Autodesk Fusion 360 part; units mm, degrees
(part 10 of 11)
  spline S69 degree 5 poles (7.9623, -22.9033) (7.9606, -22.9006) (7.9574, -22.8954) (7.9525, -22.8875) (7.9459, -22.8771) (7.9377, -22.8641) (7.9294, -22.8512) (7.9211, -22.8383) (7.9127, -22.8255) (7.9043, -22.8127) (7.8959, -22.8) (7.8874, -22.7874) (7.8788, -22.7748) (7.8702, -22.7623) (7.8616, -22.7498) (7.8529, -22.7374) (7.8442, -22.725) (7.8354, -22.7128) (7.8266, -22.7005) (7.8178, -22.6884) (7.8089, -22.6763) (7.7999, -22.6643) (7.7909, -22.6523) (7.7819, -22.6404) (7.7728, -22.6286) (7.7637, -22.6168) (7.7545, -22.6051) (7.7453, -22.5935) (7.7361, -22.5819) (7.7268, -22.5704) (7.7174, -22.559) (7.708, -22.5476) (7.6986, -22.5363) (7.6891, -22.5251) (7.6795, -22.5139) (7.6699, -22.5029) (7.6603, -22.4919) (7.6506, -22.481) (7.6409, -22.4701) (7.6311, -22.4593) (7.6213, -22.4486) (7.6114, -22.438) (7.6015, -22.4275) (7.5915, -22.417) (7.5815, -22.4067) (7.5715, -22.3964) (7.5613, -22.3862) (7.5512, -22.376) (7.5409, -22.366) (7.5307, -22.3561) (7.5204, -22.3462) (7.51, -22.3365) (7.4995, -22.3268) (7.489, -22.3173) (7.4785, -22.3078) (7.4679, -22.2984) (7.4572, -22.2892) (7.4465, -22.28) (7.4358, -22.2709) (7.4249, -22.262) (7.4141, -22.2531) (7.4031, -22.2445) (7.392, -22.236) (7.3809, -22.2276) (7.3696, -22.2194) (7.3584, -22.2113) (7.347, -22.2033) (7.3357, -22.1953) (7.3243, -22.1875) (7.3127, -22.18) (7.301, -22.1727) (7.2915, -22.1673) (7.2842, -22.1635) (7.2793, -22.161) (7.2768, -22.1599) knots -1 -1 -1 -1 -1 -1 -0.98571429 -0.97142857 -0.95714286 -0.94285714 -0.92857143 -0.91428571 -0.9 -0.88571429 -0.87142857 -0.85714286 -0.84285714 -0.82857143 -0.81428571 -0.8 -0.78571429 -0.77142857 -0.75714286 -0.74285714 -0.72857143 -0.71428571 -0.7 -0.68571429 -0.67142857 -0.65714286 -0.64285714 -0.62857143 -0.61428571 -0.6 -0.58571429 -0.57142857 -0.55714286 -0.54285714 -0.52857143 -0.51428571 -0.5 -0.48571429 -0.47142857 -0.45714286 -0.44285714 -0.42857143 -0.41428571 -0.4 -0.38571429 -0.37142857 -0.35714286 -0.34285714 -0.32857143 -0.31428571 -0.3 -0.28571429 -0.27142857 -0.25714286 -0.24285714 -0.22857143 -0.21428571 -0.2 -0.18571429 -0.17142857 -0.15714286 -0.14285714 -0.12857143 -0.11428571 -0.1 -0.08571429 -0.07142857 -0.05714286 -0.04285714 -0.02857143 -0.01428571 0 0 0 0 0 0
  line L77 (7.2768, -22.1599) -> (7.215, -22.1303)
  arc A147 (7.0927, -21.8068) -> (7.215, -22.1303) centre (7.3228, -21.9048) ccw
  arc A148 (7.0927, -21.8068) -> (7.1368, -21.7004) centre (1.6741, -19.5) ccw
  arc A149 (7.452, -21.558) -> (7.1368, -21.7004) centre (7.3687, -21.7938) ccw
  line L78 (7.452, -21.558) -> (7.5166, -21.5809)
  spline S70 degree 5 poles (7.5166, -21.5809) (7.5192, -21.5818) (7.5244, -21.5835) (7.5323, -21.586) (7.5429, -21.5889) (7.5563, -21.5921) (7.5698, -21.5949) (7.5834, -21.5974) (7.597, -21.5998) (7.6107, -21.6022) (7.6244, -21.6044) (7.6381, -21.6066) (7.6519, -21.6085) (7.6657, -21.6103) (7.6796, -21.612) (7.6936, -21.6134) (7.7076, -21.6147) (7.7216, -21.6159) (7.7356, -21.617) (7.7497, -21.618) (7.7638, -21.6189) (7.778, -21.6197) (7.7922, -21.6203) (7.8064, -21.6209) (7.8206, -21.6213) (7.8349, -21.6217) (7.8492, -21.6219) (7.8635, -21.622) (7.8778, -21.622) (7.8922, -21.622) (7.9066, -21.6218) (7.921, -21.6216) (7.9355, -21.6212) (7.9499, -21.6208) (7.9644, -21.6203) (7.9789, -21.6197) (7.9935, -21.619) (8.008, -21.6182) (8.0226, -21.6173) (8.0372, -21.6163) (8.0518, -21.6153) (8.0664, -21.6141) (8.081, -21.6129) (8.0957, -21.6116) (8.1104, -21.6102) (8.1251, -21.6088) (8.1398, -21.6072) (8.1545, -21.6056) (8.1693, -21.6039) (8.184, -21.6021) (8.1988, -21.6002) (8.2136, -21.5983) (8.2284, -21.5962) (8.2432, -21.5941) (8.258, -21.5919) (8.2729, -21.5897) (8.2877, -21.5874) (8.3026, -21.5849) (8.3175, -21.5825) (8.3324, -21.5799) (8.3473, -21.5773) (8.3622, -21.5745) (8.3771, -21.5718) (8.3921, -21.5689) (8.407, -21.566) (8.422, -21.563) (8.437, -21.5599) (8.4519, -21.5567) (8.4669, -21.5535) (8.4819, -21.5502) (8.4969, -21.5469) (8.5089, -21.5441) (8.518, -21.542) (8.524, -21.5406) (8.527, -21.5399) knots 0 0 0 0 0 0 0.01428571 0.02857143 0.04285714 0.05714286 0.07142857 0.08571429 0.1 0.11428571 0.12857143 0.14285714 0.15714286 0.17142857 0.18571429 0.2 0.21428571 0.22857143 0.24285714 0.25714286 0.27142857 0.28571429 0.3 0.31428571 0.32857143 0.34285714 0.35714286 0.37142857 0.38571429 0.4 0.41428571 0.42857143 0.44285714 0.45714286 0.47142857 0.48571429 0.5 0.51428571 0.52857143 0.54285714 0.55714286 0.57142857 0.58571429 0.6 0.61428571 0.62857143 0.64285714 0.65714286 0.67142857 0.68571429 0.7 0.71428571 0.72857143 0.74285714 0.75714286 0.77142857 0.78571429 0.8 0.81428571 0.82857143 0.84285714 0.85714286 0.87142857 0.88571429 0.9 0.91428571 0.92857143 0.94285714 0.95714286 0.97142857 0.98571429 1 1 1 1 1 1
  arc A150 (8.527, -21.5399) -> (8.6288, -21.1598) centre (1.6741, -19.5) ccw
  spline S71 degree 5 poles (8.6288, -21.1598) (8.6266, -21.1577) (8.6221, -21.1535) (8.6153, -21.1471) (8.6063, -21.1388) (8.595, -21.1283) (8.5836, -21.118) (8.5723, -21.1077) (8.5609, -21.0975) (8.5494, -21.0873) (8.538, -21.0773) (8.5265, -21.0672) (8.515, -21.0573) (8.5034, -21.0474) (8.4919, -21.0376) (8.4803, -21.0279) (8.4687, -21.0182) (8.457, -21.0086) (8.4454, -20.9991) (8.4337, -20.9896) (8.4219, -20.9803) (8.4102, -20.971) (8.3984, -20.9617) (8.3866, -20.9526) (8.3748, -20.9435) (8.3629, -20.9345) (8.351, -20.9256) (8.3391, -20.9167) (8.3272, -20.9079) (8.3152, -20.8992) (8.3032, -20.8906) (8.2912, -20.8821) (8.2791, -20.8736) (8.2671, -20.8652) (8.255, -20.8569) (8.2428, -20.8487) (8.2307, -20.8406) (8.2185, -20.8325) (8.2063, -20.8246) (8.1941, -20.8167) (8.1818, -20.8089) (8.1695, -20.8012) (8.1572, -20.7936) (8.1449, -20.7861) (8.1325, -20.7787) (8.1201, -20.7713) (8.1077, -20.7641) (8.0953, -20.757) (8.0828, -20.7499) (8.0703, -20.743) (8.0578, -20.7361) (8.0453, -20.7294) (8.0327, -20.7228) (8.0201, -20.7162) (8.0074, -20.7099) (7.9948, -20.7036) (7.9821, -20.6974) (7.9694, -20.6913) (7.9566, -20.6853) (7.9438, -20.6794) (7.931, -20.6737) (7.9182, -20.6682) (7.9053, -20.6628) (7.8924, -20.6577) (7.8794, -20.6526) (7.8664, -20.6477) (7.8534, -20.6429) (7.8404, -20.6382) (7.8273, -20.6336) (7.8142, -20.6293) (7.8011, -20.6253) (7.7904, -20.6225) (7.7824, -20.6207) (7.777, -20.6197) (7.7743, -20.6192) knots -1 -1 -1 -1 -1 -1 -0.98571429 -0.97142857 -0.95714286 -0.94285714 -0.92857143 -0.91428571 -0.9 -0.88571429 -0.87142857 -0.85714286 -0.84285714 -0.82857143 -0.81428571 -0.8 -0.78571429 -0.77142857 -0.75714286 -0.74285714 -0.72857143 -0.71428571 -0.7 -0.68571429 -0.67142857 -0.65714286 -0.64285714 -0.62857143 -0.61428571 -0.6 -0.58571429 -0.57142857 -0.55714286 -0.54285714 -0.52857143 -0.51428571 -0.5 -0.48571429 -0.47142857 -0.45714286 -0.44285714 -0.42857143 -0.41428571 -0.4 -0.38571429 -0.37142857 -0.35714286 -0.34285714 -0.32857143 -0.31428571 -0.3 -0.28571429 -0.27142857 -0.25714286 -0.24285714 -0.22857143 -0.21428571 -0.2 -0.18571429 -0.17142857 -0.15714286 -0.14285714 -0.12857143 -0.11428571 -0.1 -0.08571429 -0.07142857 -0.05714286 -0.04285714 -0.02857143 -0.01428571 0 0 0 0 0 0
  line L79 (7.7743, -20.6192) -> (7.707, -20.6066)
  arc A151 (7.5052, -20.3258) -> (7.707, -20.6066) centre (7.7527, -20.3608) ccw
  arc A152 (7.5052, -20.3258) -> (7.5202, -20.2115) centre (1.6741, -19.5) ccw
  arc A153 (7.7878, -19.9925) -> (7.5202, -20.2115) centre (7.7684, -20.2417) ccw
  line L80 (7.7878, -19.9925) -> (7.8561, -19.9978)
  spline S72 degree 5 poles (7.8561, -19.9978) (7.8588, -19.998) (7.8643, -19.9984) (7.8726, -19.9987) (7.8835, -19.9988) (7.8973, -19.9984) (7.9111, -19.9976) (7.9249, -19.9965) (7.9387, -19.9954) (7.9525, -19.9941) (7.9663, -19.9927) (7.9801, -19.9912) (7.9939, -19.9895) (8.0078, -19.9877) (8.0216, -19.9857) (8.0355, -19.9835) (8.0493, -19.9811) (8.0632, -19.9786) (8.077, -19.976) (8.0909, -19.9733) (8.1048, -19.9705) (8.1186, -19.9676) (8.1325, -19.9646) (8.1463, -19.9615) (8.1602, -19.9582) (8.1741, -19.9548) (8.188, -19.9514) (8.2018, -19.9478) (8.2157, -19.9441) (8.2295, -19.9403) (8.2434, -19.9364) (8.2573, -19.9325) (8.2711, -19.9284) (8.285, -19.9242) (8.2989, -19.92) (8.3127, -19.9156) (8.3266, -19.9112) (8.3404, -19.9067) (8.3542, -19.902) (8.3681, -19.8973) (8.3819, -19.8925) (8.3958, -19.8877) (8.4096, -19.8827) (8.4234, -19.8776) (8.4372, -19.8725) (8.451, -19.8673) (8.4649, -19.862) (8.4787, -19.8566) (8.4925, -19.8511) (8.5063, -19.8456) (8.52, -19.8399) (8.5338, -19.8342) (8.5476, -19.8284) (8.5614, -19.8226) (8.5751, -19.8166) (8.5889, -19.8106) (8.6026, -19.8045) (8.6164, -19.7983) (8.6301, -19.7921) (8.6438, -19.7857) (8.6575, -19.7793) (8.6712, -19.7729) (8.6849, -19.7663) (8.6986, -19.7597) (8.7123, -19.753) (8.726, -19.7462) (8.7397, -19.7394) (8.7533, -19.7324) (8.767, -19.7254) (8.7806, -19.7184) (8.7942, -19.7113) (8.8051, -19.7055) (8.8133, -19.7011) (8.8187, -19.6982) (8.8214, -19.6968) knots 0 0 0 0 0 0 0.01428571 0.02857143 0.04285714 0.05714286 0.07142857 0.08571429 0.1 0.11428571 0.12857143 0.14285714 0.15714286 0.17142857 0.18571429 0.2 0.21428571 0.22857143 0.24285714 0.25714286 0.27142857 0.28571429 0.3 0.31428571 0.32857143 0.34285714 0.35714286 0.37142857 0.38571429 0.4 0.41428571 0.42857143 0.44285714 0.45714286 0.47142857 0.48571429 0.5 0.51428571 0.52857143 0.54285714 0.55714286 0.57142857 0.58571429 0.6 0.61428571 0.62857143 0.64285714 0.65714286 0.67142857 0.68571429 0.7 0.71428571 0.72857143 0.74285714 0.75714286 0.77142857 0.78571429 0.8 0.81428571 0.82857143 0.84285714 0.85714286 0.87142857 0.88571429 0.9 0.91428571 0.92857143 0.94285714 0.95714286 0.97142857 0.98571429 1 1 1 1 1 1
  arc A154 (8.8214, -19.6968) -> (8.8214, -19.3032) centre (1.6741, -19.5) ccw
  spline S73 degree 5 poles (8.8214, -19.3032) (8.8187, -19.3018) (8.8133, -19.2989) (8.8051, -19.2945) (8.7942, -19.2887) (8.7806, -19.2816) (8.767, -19.2746) (8.7533, -19.2676) (8.7397, -19.2606) (8.726, -19.2538) (8.7123, -19.247) (8.6986, -19.2403) (8.6849, -19.2337) (8.6712, -19.2271) (8.6575, -19.2207) (8.6438, -19.2143) (8.6301, -19.2079) (8.6164, -19.2017) (8.6026, -19.1955) (8.5889, -19.1894) (8.5751, -19.1834) (8.5614, -19.1774) (8.5476, -19.1716) (8.5338, -19.1658) (8.52, -19.1601) (8.5063, -19.1544) (8.4925, -19.1489) (8.4787, -19.1434) (8.4649, -19.138) (8.451, -19.1327) (8.4372, -19.1275) (8.4234, -19.1224) (8.4096, -19.1173) (8.3958, -19.1123) (8.3819, -19.1075) (8.3681, -19.1027) (8.3542, -19.098) (8.3404, -19.0933) (8.3266, -19.0888) (8.3127, -19.0844) (8.2989, -19.08) (8.285, -19.0758) (8.2711, -19.0716) (8.2573, -19.0675) (8.2434, -19.0636) (8.2295, -19.0597) (8.2157, -19.0559) (8.2018, -19.0522) (8.188, -19.0486) (8.1741, -19.0452) (8.1602, -19.0418) (8.1463, -19.0385) (8.1325, -19.0354) (8.1186, -19.0324) (8.1048, -19.0295) (8.0909, -19.0267) (8.077, -19.024) (8.0632, -19.0214) (8.0493, -19.0189) (8.0355, -19.0165) (8.0216, -19.0143) (8.0078, -19.0123) (7.9939, -19.0105) (7.9801, -19.0088) (7.9663, -19.0073) (7.9525, -19.0059) (7.9387, -19.0046) (7.9249, -19.0035) (7.9111, -19.0024) (7.8973, -19.0016) (7.8835, -19.0012) (7.8726, -19.0013) (7.8643, -19.0016) (7.8588, -19.002) (7.8561, -19.0022) knots -1 -1 -1 -1 -1 -1 -0.98571429 -0.97142857 -0.95714286 -0.94285714 -0.92857143 -0.91428571 -0.9 -0.88571429 -0.87142857 -0.85714286 -0.84285714 -0.82857143 -0.81428571 -0.8 -0.78571429 -0.77142857 -0.75714286 -0.74285714 -0.72857143 -0.71428571 -0.7 -0.68571429 -0.67142857 -0.65714286 -0.64285714 -0.62857143 -0.61428571 -0.6 -0.58571429 -0.57142857 -0.55714286 -0.54285714 -0.52857143 -0.51428571 -0.5 -0.48571429 -0.47142857 -0.45714286 -0.44285714 -0.42857143 -0.41428571 -0.4 -0.38571429 -0.37142857 -0.35714286 -0.34285714 -0.32857143 -0.31428571 -0.3 -0.28571429 -0.27142857 -0.25714286 -0.24285714 -0.22857143 -0.21428571 -0.2 -0.18571429 -0.17142857 -0.15714286 -0.14285714 -0.12857143 -0.11428571 -0.1 -0.08571429 -0.07142857 -0.05714286 -0.04285714 -0.02857143 -0.01428571 0 0 0 0 0 0
  line L81 (7.8561, -19.0022) -> (7.7878, -19.0075)
  arc A155 (7.5202, -18.7885) -> (7.7878, -19.0075) centre (7.7684, -18.7583) ccw
  arc A156 (7.5202, -18.7885) -> (7.5052, -18.6742) centre (1.6741, -19.5) ccw
  arc A157 (7.707, -18.3934) -> (7.5052, -18.6742) centre (7.7527, -18.6392) ccw
  line L82 (7.707, -18.3934) -> (7.7743, -18.3808)
  spline S74 degree 5 poles (7.7743, -18.3808) (7.777, -18.3803) (7.7824, -18.3793) (7.7904, -18.3775) (7.8011, -18.3747) (7.8142, -18.3707) (7.8273, -18.3664) (7.8404, -18.3618) (7.8534, -18.3571) (7.8664, -18.3523) (7.8794, -18.3474) (7.8924, -18.3423) (7.9053, -18.3372) (7.9182, -18.3318) (7.931, -18.3263) (7.9438, -18.3206) (7.9566, -18.3147) (7.9694, -18.3087) (7.9821, -18.3026) (7.9948, -18.2964) (8.0074, -18.2901) (8.0201, -18.2838) (8.0327, -18.2772) (8.0453, -18.2706) (8.0578, -18.2639) (8.0703, -18.257) (8.0828, -18.2501) (8.0953, -18.243) (8.1077, -18.2359) (8.1201, -18.2287) (8.1325, -18.2213) (8.1449, -18.2139) (8.1572, -18.2064) (8.1695, -18.1988) (8.1818, -18.1911) (8.1941, -18.1833) (8.2063, -18.1754) (8.2185, -18.1675) (8.2307, -18.1594) (8.2428, -18.1513) (8.255, -18.1431) (8.2671, -18.1348) (8.2791, -18.1264) (8.2912, -18.1179) (8.3032, -18.1094) (8.3152, -18.1008) (8.3272, -18.0921) (8.3391, -18.0833) (8.351, -18.0744) (8.3629, -18.0655) (8.3748, -18.0565) (8.3866, -18.0474) (8.3984, -18.0383) (8.4102, -18.029) (8.4219, -18.0197) (8.4337, -18.0104) (8.4454, -18.0009) (8.457, -17.9914) (8.4687, -17.9818) (8.4803, -17.9721) (8.4919, -17.9624) (8.5034, -17.9526) (8.515, -17.9427) (8.5265, -17.9328) (8.538, -17.9227) (8.5494, -17.9127) (8.5609, -17.9025) (8.5723, -17.8923) (8.5836, -17.882) (8.595, -17.8717) (8.6063, -17.8612) (8.6153, -17.8529) (8.6221, -17.8465) (8.6266, -17.8423) (8.6288, -17.8402) knots 0 0 0 0 0 0 0.01428571 0.02857143 0.04285714 0.05714286 0.07142857 0.08571429 0.1 0.11428571 0.12857143 0.14285714 0.15714286 0.17142857 0.18571429 0.2 0.21428571 0.22857143 0.24285714 0.25714286 0.27142857 0.28571429 0.3 0.31428571 0.32857143 0.34285714 0.35714286 0.37142857 0.38571429 0.4 0.41428571 0.42857143 0.44285714 0.45714286 0.47142857 0.48571429 0.5 0.51428571 0.52857143 0.54285714 0.55714286 0.57142857 0.58571429 0.6 0.61428571 0.62857143 0.64285714 0.65714286 0.67142857 0.68571429 0.7 0.71428571 0.72857143 0.74285714 0.75714286 0.77142857 0.78571429 0.8 0.81428571 0.82857143 0.84285714 0.85714286 0.87142857 0.88571429 0.9 0.91428571 0.92857143 0.94285714 0.95714286 0.97142857 0.98571429 1 1 1 1 1 1
  arc A158 (8.6288, -17.8402) -> (8.527, -17.4601) centre (1.6741, -19.5) ccw
  spline S75 degree 5 poles (8.527, -17.4601) (8.524, -17.4594) (8.518, -17.458) (8.5089, -17.4559) (8.4969, -17.4531) (8.4819, -17.4498) (8.4669, -17.4465) (8.4519, -17.4433) (8.437, -17.4401) (8.422, -17.437) (8.407, -17.434) (8.3921, -17.4311) (8.3771, -17.4282) (8.3622, -17.4255) (8.3473, -17.4227) (8.3324, -17.4201) (8.3175, -17.4175) (8.3026, -17.4151) (8.2877, -17.4126) (8.2729, -17.4103) (8.258, -17.4081) (8.2432, -17.4059) (8.2284, -17.4038) (8.2136, -17.4017) (8.1988, -17.3998) (8.184, -17.3979) (8.1693, -17.3961) (8.1545, -17.3944) (8.1398, -17.3928) (8.1251, -17.3912) (8.1104, -17.3898) (8.0957, -17.3884) (8.081, -17.3871) (8.0664, -17.3859) (8.0518, -17.3847) (8.0372, -17.3837) (8.0226, -17.3827) (8.008, -17.3818) (7.9935, -17.381) (7.9789, -17.3803) (7.9644, -17.3797) (7.9499, -17.3792) (7.9355, -17.3788) (7.921, -17.3784) (7.9066, -17.3782) (7.8922, -17.378) (7.8778, -17.378) (7.8635, -17.378) (7.8492, -17.3781) (7.8349, -17.3783) (7.8206, -17.3787) (7.8064, -17.3791) (7.7922, -17.3797) (7.778, -17.3803) (7.7638, -17.3811) (7.7497, -17.382) (7.7356, -17.383) (7.7216, -17.3841) (7.7076, -17.3853) (7.6936, -17.3866) (7.6796, -17.388) (7.6657, -17.3897) (7.6519, -17.3915) (7.6381, -17.3934) (7.6244, -17.3956) (7.6107, -17.3978) (7.597, -17.4002) (7.5834, -17.4026) (7.5698, -17.4051) (7.5563, -17.4079) (7.5429, -17.4111) (7.5323, -17.414) (7.5244, -17.4165) (7.5192, -17.4182) (7.5166, -17.4191) knots -1 -1 -1 -1 -1 -1 -0.98571429 -0.97142857 -0.95714286 -0.94285714 -0.92857143 -0.91428571 -0.9 -0.88571429 -0.87142857 -0.85714286 -0.84285714 -0.82857143 -0.81428571 -0.8 -0.78571429 -0.77142857 -0.75714286 -0.74285714 -0.72857143 -0.71428571 -0.7 -0.68571429 -0.67142857 -0.65714286 -0.64285714 -0.62857143 -0.61428571 -0.6 -0.58571429 -0.57142857 -0.55714286 -0.54285714 -0.52857143 -0.51428571 -0.5 -0.48571429 -0.47142857 -0.45714286 -0.44285714 -0.42857143 -0.41428571 -0.4 -0.38571429 -0.37142857 -0.35714286 -0.34285714 -0.32857143 -0.31428571 -0.3 -0.28571429 -0.27142857 -0.25714286 -0.24285714 -0.22857143 -0.21428571 -0.2 -0.18571429 -0.17142857 -0.15714286 -0.14285714 -0.12857143 -0.11428571 -0.1 -0.08571429 -0.07142857 -0.05714286 -0.04285714 -0.02857143 -0.01428571 0 0 0 0 0 0
  line L83 (7.5166, -17.4191) -> (7.452, -17.442)
  arc A159 (7.1368, -17.2996) -> (7.452, -17.442) centre (7.3687, -17.2062) ccw
  arc A160 (7.1368, -17.2996) -> (7.0927, -17.1932) centre (1.6741, -19.5) ccw
  arc A161 (7.215, -16.8697) -> (7.0927, -17.1932) centre (7.3228, -17.0952) ccw
  line L84 (7.215, -16.8697) -> (7.2768, -16.8401)
  spline S76 degree 5 poles (7.2768, -16.8401) (7.2793, -16.839) (7.2842, -16.8365) (7.2915, -16.8327) (7.301, -16.8273) (7.3127, -16.82) (7.3243, -16.8125) (7.3357, -16.8047) (7.347, -16.7967) (7.3584, -16.7887) (7.3696, -16.7806) (7.3809, -16.7724) (7.392, -16.764) (7.4031, -16.7555) (7.4141, -16.7469) (7.4249, -16.738) (7.4358, -16.7291) (7.4465, -16.72) (7.4572, -16.7108) (7.4679, -16.7016) (7.4785, -16.6922) (7.489, -16.6827) (7.4995, -16.6732) (7.51, -16.6635) (7.5204, -16.6538) (7.5307, -16.6439) (7.5409, -16.634) (7.5512, -16.624) (7.5613, -16.6138) (7.5715, -16.6036) (7.5815, -16.5933) (7.5915, -16.583) (7.6015, -16.5725) (7.6114, -16.562) (7.6213, -16.5514) (7.6311, -16.5407) (7.6409, -16.5299) (7.6506, -16.5191) (7.6603, -16.5081) (7.6699, -16.4971) (7.6795, -16.4861) (7.6891, -16.4749) (7.6986, -16.4637) (7.708, -16.4524) (7.7174, -16.441) (7.7268, -16.4296) (7.7361, -16.4181) (7.7453, -16.4065) (7.7545, -16.3949) (7.7637, -16.3832) (7.7728, -16.3714) (7.7819, -16.3596) (7.7909, -16.3477) (7.7999, -16.3357) (7.8089, -16.3237) (7.8178, -16.3116) (7.8266, -16.2995) (7.8354, -16.2872) (7.8442, -16.275) (7.8529, -16.2626) (7.8616, -16.2502) (7.8702, -16.2378) (7.8788, -16.2252) (7.8874, -16.2126) (7.8959, -16.2) (7.9043, -16.1873) (7.9127, -16.1745) (7.9211, -16.1617) (7.9294, -16.1488) (7.9377, -16.1359) (7.9459, -16.1229) (7.9525, -16.1125) (7.9574, -16.1046) (7.9606, -16.0994) (7.9623, -16.0967) knots 0 0 0 0 0 0 0.01428571 0.02857143 0.04285714 0.05714286 0.07142857 0.08571429 0.1 0.11428571 0.12857143 0.14285714 0.15714286 0.17142857 0.18571429 0.2 0.21428571 0.22857143 0.24285714 0.25714286 0.27142857 0.28571429 0.3 0.31428571 0.32857143 0.34285714 0.35714286 0.37142857 0.38571429 0.4 0.41428571 0.42857143 0.44285714 0.45714286 0.47142857 0.48571429 0.5 0.51428571 0.52857143 0.54285714 0.55714286 0.57142857 0.58571429 0.6 0.61428571 0.62857143 0.64285714 0.65714286 0.67142857 0.68571429 0.7 0.71428571 0.72857143 0.74285714 0.75714286 0.77142857 0.78571429 0.8 0.81428571 0.82857143 0.84285714 0.85714286 0.87142857 0.88571429 0.9 0.91428571 0.92857143 0.94285714 0.95714286 0.97142857 0.98571429 1 1 1 1 1 1
  arc A162 (7.9623, -16.0967) -> (7.7655, -15.756) centre (1.6741, -19.5) ccw
  spline S77 degree 5 poles (7.7655, -15.756) (7.7624, -15.7561) (7.7562, -15.7562) (7.747, -15.7566) (7.7347, -15.757) (7.7193, -15.7576) (7.704, -15.7583) (7.6887, -15.7591) (7.6734, -15.76) (7.6581, -15.7609) (7.6429, -15.7618) (7.6277, -15.7629) (7.6125, -15.764) (7.5974, -15.7651) (7.5823, -15.7664) (7.5672, -15.7677) (7.5521, -15.7691) (7.5371, -15.7705) (7.5221, -15.772) (7.5072, -15.7736) (7.4923, -15.7753) (7.4774, -15.777) (7.4625, -15.7788) (7.4477, -15.7807) (7.4329, -15.7827) (7.4181, -15.7847) (7.4034, -15.7868) (7.3887, -15.7889) (7.3741, -15.7912) (7.3595, -15.7935) (7.3449, -15.7959) (7.3304, -15.7983) (7.3159, -15.8009) (7.3014, -15.8035) (7.287, -15.8062) (7.2726, -15.8089) (7.2583, -15.8118) (7.244, -15.8147) (7.2297, -15.8177) (7.2155, -15.8208) (7.2013, -15.8239) (7.1872, -15.8272) (7.1731, -15.8305) (7.1591, -15.8339) (7.1451, -15.8374) (7.1311, -15.841) (7.1172, -15.8446) (7.1034, -15.8484) (7.0896, -15.8522) (7.0758, -15.8561) (7.0621, -15.8601) (7.0485, -15.8642) (7.0349, -15.8685) (7.0214, -15.8728) (7.0079, -15.8772) (6.9945, -15.8817) (6.9812, -15.8863) (6.9679, -15.891) (6.9546, -15.8957) (6.9415, -15.9006) (6.9284, -15.9057) (6.9154, -15.9108) (6.9025, -15.9162) (6.8897, -15.9216) (6.877, -15.9272) (6.8643, -15.933) (6.8517, -15.9388) (6.8391, -15.9446) (6.8267, -15.9506) (6.8144, -15.9568) (6.8022, -15.9633) (6.7928, -15.9689) (6.7858, -15.9733) (6.7812, -15.9763) (6.779, -15.9779) knots -1 -1 -1 -1 -1 -1 -0.98571429 -0.97142857 -0.95714286 -0.94285714 -0.92857143 -0.91428571 -0.9 -0.88571429 -0.87142857 -0.85714286 -0.84285714 -0.82857143 -0.81428571 -0.8 -0.78571429 -0.77142857 -0.75714286 -0.74285714 -0.72857143 -0.71428571 -0.7 -0.68571429 -0.67142857 -0.65714286 -0.64285714 -0.62857143 -0.61428571 -0.6 -0.58571429 -0.57142857 -0.55714286 -0.54285714 -0.52857143 -0.51428571 -0.5 -0.48571429 -0.47142857 -0.45714286 -0.44285714 -0.42857143 -0.41428571 -0.4 -0.38571429 -0.37142857 -0.35714286 -0.34285714 -0.32857143 -0.31428571 -0.3 -0.28571429 -0.27142857 -0.25714286 -0.24285714 -0.22857143 -0.21428571 -0.2 -0.18571429 -0.17142857 -0.15714286 -0.14285714 -0.12857143 -0.11428571 -0.1 -0.08571429 -0.07142857 -0.05714286 -0.04285714 -0.02857143 -0.01428571 0 0 0 0 0 0
  line L85 (6.779, -15.9779) -> (6.7225, -16.0167)
  arc A163 (6.3812, -15.9608) -> (6.7225, -16.0167) centre (6.581, -15.8105) ccw
  arc A164 (6.3812, -15.9608) -> (6.3111, -15.8693) centre (1.6741, -19.5) ccw
  arc A165 (6.3454, -15.5252) -> (6.3111, -15.8693) centre (6.5079, -15.7152) ccw
  line L86 (6.3454, -15.5252) -> (6.3975, -15.4807)
  spline S78 degree 5 poles (6.3975, -15.4807) (6.3995, -15.4789) (6.4037, -15.4753) (6.4097, -15.4697) (6.4176, -15.462) (6.427, -15.452) (6.4362, -15.4417) (6.4452, -15.4312) (6.4541, -15.4206) (6.4629, -15.4099) (6.4717, -15.3992) (6.4805, -15.3883) (6.4891, -15.3774) (6.4975, -15.3663) (6.5059, -15.3551) (6.5141, -15.3437) (6.5223, -15.3323) (6.5303, -15.3207) (6.5383, -15.3091) (6.5462, -15.2974) (6.554, -15.2856) (6.5617, -15.2737) (6.5694, -15.2618) (6.577, -15.2498) (6.5845, -15.2377) (6.5919, -15.2255) (6.5993, -15.2132) (6.6065, -15.2009) (6.6137, -15.1885) (6.6209, -15.176) (6.6279, -15.1634) (6.6349, -15.1508) (6.6419, -15.1382) (6.6487, -15.1254) (6.6555, -15.1126) (6.6622, -15.0997) (6.6689, -15.0868) (6.6755, -15.0738) (6.682, -15.0607) (6.6884, -15.0476) (6.6948, -15.0344) (6.7012, -15.0212) (6.7074, -15.0079) (6.7136, -14.9946) (6.7198, -14.9812) (6.7258, -14.9677) (6.7319, -14.9542) (6.7378, -14.9406) (6.7437, -14.927) (6.7495, -14.9133) (6.7553, -14.8996) (6.761, -14.8858) (6.7666, -14.872) (6.7722, -14.8581) (6.7778, -14.8442) (6.7832, -14.8302) (6.7886, -14.8161) (6.794, -14.8021) (6.7993, -14.7879) (6.8045, -14.7737) (6.8097, -14.7595) (6.8148, -14.7452) (6.8198, -14.7309) (6.8248, -14.7166) (6.8298, -14.7021) (6.8346, -14.6877) (6.8395, -14.6732) (6.8442, -14.6586) (6.8489, -14.644) (6.8536, -14.6294) (6.8582, -14.6147) (6.8618, -14.6029) (6.8645, -14.5941) (6.8663, -14.5882) (6.8672, -14.5852) knots 0 0 0 0 0 0 0.01428571 0.02857143 0.04285714 0.05714286 0.07142857 0.08571429 0.1 0.11428571 0.12857143 0.14285714 0.15714286 0.17142857 0.18571429 0.2 0.21428571 0.22857143 0.24285714 0.25714286 0.27142857 0.28571429 0.3 0.31428571 0.32857143 0.34285714 0.35714286 0.37142857 0.38571429 0.4 0.41428571 0.42857143 0.44285714 0.45714286 0.47142857 0.48571429 0.5 0.51428571 0.52857143 0.54285714 0.55714286 0.57142857 0.58571429 0.6 0.61428571 0.62857143 0.64285714 0.65714286 0.67142857 0.68571429 0.7 0.71428571 0.72857143 0.74285714 0.75714286 0.77142857 0.78571429 0.8 0.81428571 0.82857143 0.84285714 0.85714286 0.87142857 0.88571429 0.9 0.91428571 0.92857143 0.94285714 0.95714286 0.97142857 0.98571429 1 1 1 1 1 1
  arc A166 (6.8672, -14.5852) -> (6.5889, -14.307) centre (1.6741, -19.5) ccw
  spline S79 degree 5 poles (6.5889, -14.307) (6.586, -14.3079) (6.58, -14.3097) (6.5712, -14.3123) (6.5594, -14.316) (6.5447, -14.3206) (6.5301, -14.3252) (6.5155, -14.3299) (6.501, -14.3347) (6.4865, -14.3395) (6.472, -14.3444) (6.4576, -14.3493) (6.4432, -14.3543) (6.4289, -14.3594) (6.4146, -14.3645) (6.4004, -14.3696) (6.3862, -14.3749) (6.3721, -14.3802) (6.358, -14.3855) (6.344, -14.3909) (6.33, -14.3964) (6.3161, -14.4019) (6.3022, -14.4075) (6.2883, -14.4131) (6.2746, -14.4188) (6.2608, -14.4246) (6.2471, -14.4304) (6.2335, -14.4363) (6.22, -14.4423) (6.2064, -14.4483) (6.193, -14.4544) (6.1796, -14.4605) (6.1662, -14.4667) (6.1529, -14.473) (6.1397, -14.4793) (6.1265, -14.4857) (6.1134, -14.4922) (6.1003, -14.4987) (6.0873, -14.5053) (6.0744, -14.5119) (6.0615, -14.5186) (6.0487, -14.5254) (6.036, -14.5323) (6.0233, -14.5392) (6.0107, -14.5462) (5.9982, -14.5533) (5.9857, -14.5604) (5.9733, -14.5676) (5.9609, -14.5749) (5.9487, -14.5822) (5.9365, -14.5896) (5.9244, -14.5971) (5.9123, -14.6047) (5.9004, -14.6124) (5.8885, -14.6201) (5.8768, -14.628) (5.8651, -14.6359) (5.8534, -14.6438) (5.8419, -14.6519) (5.8304, -14.66) (5.8191, -14.6682) (5.8078, -14.6766) (5.7968, -14.6851) (5.7858, -14.6937) (5.775, -14.7024) (5.7642, -14.7112) (5.7536, -14.7201) (5.743, -14.729) (5.7325, -14.738) (5.7222, -14.7471) (5.7121, -14.7566) (5.7044, -14.7644) (5.6988, -14.7705) (5.6952, -14.7746) (5.6934, -14.7767) knots -1 -1 -1 -1 -1 -1 -0.98571429 -0.97142857 -0.95714286 -0.94285714 -0.92857143 -0.91428571 -0.9 -0.88571429 -0.87142857 -0.85714286 -0.84285714 -0.82857143 -0.81428571 -0.8 -0.78571429 -0.77142857 -0.75714286 -0.74285714 -0.72857143 -0.71428571 -0.7 -0.68571429 -0.67142857 -0.65714286 -0.64285714 -0.62857143 -0.61428571 -0.6 -0.58571429 -0.57142857 -0.55714286 -0.54285714 -0.52857143 -0.51428571 -0.5 -0.48571429 -0.47142857 -0.45714286 -0.44285714 -0.42857143 -0.41428571 -0.4 -0.38571429 -0.37142857 -0.35714286 -0.34285714 -0.32857143 -0.31428571 -0.3 -0.28571429 -0.27142857 -0.25714286 -0.24285714 -0.22857143 -0.21428571 -0.2 -0.18571429 -0.17142857 -0.15714286 -0.14285714 -0.12857143 -0.11428571 -0.1 -0.08571429 -0.07142857 -0.05714286 -0.04285714 -0.02857143 -0.01428571 0 0 0 0 0 0
  line L87 (5.6934, -14.7767) -> (5.6489, -14.8287)
  arc A167 (5.3048, -14.8631) -> (5.6489, -14.8287) centre (5.4589, -14.6662) ccw
  arc A168 (5.3048, -14.8631) -> (5.2134, -14.7929) centre (1.6741, -19.5) ccw
  arc A169 (5.1575, -14.4516) -> (5.2134, -14.7929) centre (5.3636, -14.5931) ccw
  line L88 (5.1575, -14.4516) -> (5.1962, -14.3952)
  spline S80 degree 5 poles (5.1962, -14.3952) (5.1978, -14.3929) (5.2009, -14.3883) (5.2053, -14.3814) (5.2108, -14.3719) (5.2173, -14.3598) (5.2235, -14.3475) (5.2295, -14.335) (5.2354, -14.3224) (5.2412, -14.3098) (5.2469, -14.2972) (5.2525, -14.2845) (5.258, -14.2717) (5.2633, -14.2588) (5.2685, -14.2458) (5.2735, -14.2327) (5.2784, -14.2195) (5.2832, -14.2063) (5.2879, -14.193) (5.2924, -14.1796) (5.297, -14.1662) (5.3014, -14.1527) (5.3057, -14.1392) (5.3099, -14.1256) (5.314, -14.112) (5.318, -14.0983) (5.3219, -14.0846) (5.3258, -14.0708) (5.3295, -14.0569) (5.3332, -14.043) (5.3368, -14.0291) (5.3402, -14.0151) (5.3437, -14.001) (5.347, -13.987) (5.3502, -13.9728) (5.3534, -13.9587) (5.3565, -13.9444) (5.3595, -13.9302) (5.3624, -13.9159) (5.3652, -13.9015) (5.368, -13.8872) (5.3707, -13.8727) (5.3733, -13.8583) (5.3758, -13.8438) (5.3783, -13.8292) (5.3807, -13.8147) (5.383, -13.8) (5.3852, -13.7854) (5.3874, -13.7707) (5.3895, -13.756) (5.3915, -13.7412) (5.3934, -13.7265) (5.3953, -13.7116) (5.3971, -13.6968) (5.3988, -13.6819) (5.4005, -13.667) (5.4021, -13.652) (5.4036, -13.637) (5.4051, -13.622) (5.4064, -13.6069) (5.4078, -13.5919) (5.409, -13.5768) (5.4102, -13.5616) (5.4113, -13.5464) (5.4123, -13.5312) (5.4133, -13.516) (5.4142, -13.5008) (5.415, -13.4855) (5.4158, -13.4702) (5.4165, -13.4548) (5.4171, -13.4395) (5.4176, -13.4271) (5.4179, -13.4179) (5.4181, -13.4117) (5.4182, -13.4086) knots 0 0 0 0 0 0 0.01428571 0.02857143 0.04285714 0.05714286 0.07142857 0.08571429 0.1 0.11428571 0.12857143 0.14285714 0.15714286 0.17142857 0.18571429 0.2 0.21428571 0.22857143 0.24285714 0.25714286 0.27142857 0.28571429 0.3 0.31428571 0.32857143 0.34285714 0.35714286 0.37142857 0.38571429 0.4 0.41428571 0.42857143 0.44285714 0.45714286 0.47142857 0.48571429 0.5 0.51428571 0.52857143 0.54285714 0.55714286 0.57142857 0.58571429 0.6 0.61428571 0.62857143 0.64285714 0.65714286 0.67142857 0.68571429 0.7 0.71428571 0.72857143 0.74285714 0.75714286 0.77142857 0.78571429 0.8 0.81428571 0.82857143 0.84285714 0.85714286 0.87142857 0.88571429 0.9 0.91428571 0.92857143 0.94285714 0.95714286 0.97142857 0.98571429 1 1 1 1 1 1
  arc A170 (5.4182, -13.4086) -> (5.0774, -13.2119) centre (1.6741, -19.5) ccw
  spline S81 degree 5 poles (5.0774, -13.2119) (5.0748, -13.2135) (5.0695, -13.2168) (5.0617, -13.2217) (5.0512, -13.2282) (5.0382, -13.2364) (5.0253, -13.2447) (5.0124, -13.253) (4.9996, -13.2614) (4.9868, -13.2698) (4.9741, -13.2783) (4.9615, -13.2868) (4.9489, -13.2953) (4.9364, -13.3039) (4.9239, -13.3125) (4.9115, -13.3212) (4.8992, -13.3299) (4.8869, -13.3387) (4.8747, -13.3475) (4.8625, -13.3564) (4.8504, -13.3653) (4.8384, -13.3742) (4.8264, -13.3832) (4.8145, -13.3922) (4.8027, -13.4013) (4.7909, -13.4104) (4.7792, -13.4196) (4.7676, -13.4288) (4.756, -13.4381) (4.7445, -13.4474) (4.7331, -13.4567) (4.7217, -13.4661) (4.7104, -13.4756) (4.6992, -13.4851) (4.6881, -13.4946) (4.677, -13.5042) (4.666, -13.5138) (4.6551, -13.5235) (4.6442, -13.5332) (4.6335, -13.543) (4.6228, -13.5528) (4.6122, -13.5627) (4.6016, -13.5726) (4.5912, -13.5826) (4.5808, -13.5926) (4.5705, -13.6027) (4.5603, -13.6128) (4.5502, -13.623) (4.5402, -13.6332) (4.5302, -13.6435) (4.5204, -13.6538) (4.5106, -13.6642) (4.5009, -13.6746) (4.4914, -13.6851) (4.4819, -13.6957) (4.4726, -13.7063) (4.4633, -13.7169) (4.4541, -13.7276) (4.4451, -13.7384) (4.4361, -13.7492) (4.4273, -13.7601) (4.4186, -13.7711) (4.4101, -13.7821) (4.4017, -13.7933) (4.3935, -13.8045) (4.3854, -13.8158) (4.3774, -13.8271) (4.3695, -13.8384) (4.3617, -13.8499) (4.3541, -13.8614) (4.3469, -13.8731) (4.3414, -13.8826) (4.3376, -13.8899) (4.3352, -13.8949) (4.334, -13.8974) knots -1 -1 -1 -1 -1 -1 -0.98571429 -0.97142857 -0.95714286 -0.94285714 -0.92857143 -0.91428571 -0.9 -0.88571429 -0.87142857 -0.85714286 -0.84285714 -0.82857143 -0.81428571 -0.8 -0.78571429 -0.77142857 -0.75714286 -0.74285714 -0.72857143 -0.71428571 -0.7 -0.68571429 -0.67142857 -0.65714286 -0.64285714 -0.62857143 -0.61428571 -0.6 -0.58571429 -0.57142857 -0.55714286 -0.54285714 -0.52857143 -0.51428571 -0.5 -0.48571429 -0.47142857 -0.45714286 -0.44285714 -0.42857143 -0.41428571 -0.4 -0.38571429 -0.37142857 -0.35714286 -0.34285714 -0.32857143 -0.31428571 -0.3 -0.28571429 -0.27142857 -0.25714286 -0.24285714 -0.22857143 -0.21428571 -0.2 -0.18571429 -0.17142857 -0.15714286 -0.14285714 -0.12857143 -0.11428571 -0.1 -0.08571429 -0.07142857 -0.05714286 -0.04285714 -0.02857143 -0.01428571 0 0 0 0 0 0
  line L89 (4.334, -13.8974) -> (4.3045, -13.9592)
  arc A171 (3.981, -14.0814) -> (4.3045, -13.9592) centre (4.0789, -13.8514) ccw
  arc A172 (3.981, -14.0814) -> (3.8745, -14.0373) centre (1.6741, -19.5) ccw
  arc A173 (3.7322, -13.7221) -> (3.8745, -14.0373) centre (3.9679, -13.8054) ccw
  line L90 (3.7322, -13.7221) -> (3.755, -13.6575)
  spline S82 degree 5 poles (3.755, -13.6575) (3.7559, -13.6549) (3.7577, -13.6497) (3.7601, -13.6419) (3.7631, -13.6313) (3.7662, -13.6179) (3.769, -13.6044) (3.7716, -13.5908) (3.774, -13.5771) (3.7763, -13.5635) (3.7786, -13.5498) (3.7807, -13.536) (3.7827, -13.5222) (3.7845, -13.5084) (3.7861, -13.4945) (3.7876, -13.4806) (3.7889, -13.4666) (3.7901, -13.4525) (3.7912, -13.4385) (3.7921, -13.4244) (3.793, -13.4103) (3.7938, -13.3961) (3.7945, -13.382) (3.795, -13.3678) (3.7955, -13.3535) (3.7958, -13.3393) (3.796, -13.325) (3.7962, -13.3106) (3.7962, -13.2963) (3.7961, -13.2819) (3.796, -13.2675) (3.7957, -13.2531) (3.7954, -13.2387) (3.7949, -13.2242) (3.7944, -13.2097) (3.7938, -13.1952) (3.7931, -13.1807) (3.7923, -13.1661) (3.7914, -13.1516) (3.7905, -13.137) (3.7894, -13.1224) (3.7883, -13.1077) (3.787, -13.0931) (3.7857, -13.0784) (3.7844, -13.0638) (3.7829, -13.0491) (3.7813, -13.0344) (3.7797, -13.0196) (3.778, -13.0049) (3.7762, -12.9901) (3.7743, -12.9753) (3.7724, -12.9606) (3.7704, -12.9458) (3.7683, -12.9309) (3.7661, -12.9161) (3.7638, -12.9013) (3.7615, -12.8864) (3.7591, -12.8715) (3.7566, -12.8567) (3.754, -12.8418) (3.7514, -12.8269) (3.7487, -12.8119) (3.7459, -12.797) (3.743, -12.7821) (3.7401, -12.7671) (3.7371, -12.7522) (3.734, -12.7372) (3.7309, -12.7222) (3.7277, -12.7072) (3.7244, -12.6922) (3.721, -12.6772) (3.7183, -12.6652) (3.7162, -12.6562) (3.7148, -12.6502) (3.714, -12.6472) knots 0 0 0 0 0 0 0.01428571 0.02857143 0.04285714 0.05714286 0.07142857 0.08571429 0.1 0.11428571 0.12857143 0.14285714 0.15714286 0.17142857 0.18571429 0.2 0.21428571 0.22857143 0.24285714 0.25714286 0.27142857 0.28571429 0.3 0.31428571 0.32857143 0.34285714 0.35714286 0.37142857 0.38571429 0.4 0.41428571 0.42857143 0.44285714 0.45714286 0.47142857 0.48571429 0.5 0.51428571 0.52857143 0.54285714 0.55714286 0.57142857 0.58571429 0.6 0.61428571 0.62857143 0.64285714 0.65714286 0.67142857 0.68571429 0.7 0.71428571 0.72857143 0.74285714 0.75714286 0.77142857 0.78571429 0.8 0.81428571 0.82857143 0.84285714 0.85714286 0.87142857 0.88571429 0.9 0.91428571 0.92857143 0.94285714 0.95714286 0.97142857 0.98571429 1 1 1 1 1 1
  arc A174 (3.714, -12.6472) -> (3.3339, -12.5453) centre (1.6741, -19.5) ccw
  spline S83 degree 5 poles (3.3339, -12.5453) (3.3318, -12.5476) (3.3276, -12.5521) (3.3213, -12.5588) (3.3129, -12.5679) (3.3025, -12.5792) (3.2921, -12.5905) (3.2818, -12.6019) (3.2716, -12.6133) (3.2615, -12.6247) (3.2514, -12.6362) (3.2414, -12.6476) (3.2314, -12.6592) (3.2216, -12.6707) (3.2118, -12.6823) (3.202, -12.6938) (3.1924, -12.7055) (3.1828, -12.7171) (3.1732, -12.7288) (3.1638, -12.7405) (3.1544, -12.7522) (3.1451, -12.764) (3.1359, -12.7757) (3.1267, -12.7875) (3.1176, -12.7994) (3.1086, -12.8112) (3.0997, -12.8231) (3.0908, -12.835) (3.0821, -12.847) (3.0734, -12.8589) (3.0648, -12.8709) (3.0562, -12.883) (3.0478, -12.895) (3.0394, -12.9071) (3.0311, -12.9192) (3.0229, -12.9313) (3.0147, -12.9435) (3.0067, -12.9556) (2.9987, -12.9678) (2.9908, -12.9801) (2.9831, -12.9923) (2.9754, -13.0046) (2.9678, -13.0169) (2.9602, -13.0292) (2.9528, -13.0416) (2.9455, -13.054) (2.9382, -13.0664) (2.9311, -13.0789) (2.9241, -13.0913) (2.9171, -13.1038) (2.9103, -13.1163) (2.9035, -13.1289) (2.8969, -13.1415) (2.8904, -13.1541) (2.884, -13.1667) (2.8777, -13.1794) (2.8715, -13.1921) (2.8654, -13.2048) (2.8594, -13.2175) (2.8536, -13.2303) (2.8479, -13.2431) (2.8423, -13.256) (2.837, -13.2688) (2.8318, -13.2818) (2.8268, -13.2947) (2.8219, -13.3077) (2.817, -13.3207) (2.8123, -13.3338) (2.8077, -13.3468) (2.8034, -13.3599) (2.7994, -13.3731) (2.7967, -13.3837) (2.7949, -13.3917) (2.7938, -13.3971) (2.7933, -13.3998) knots -1 -1 -1 -1 -1 -1 -0.98571429 -0.97142857 -0.95714286 -0.94285714 -0.92857143 -0.91428571 -0.9 -0.88571429 -0.87142857 -0.85714286 -0.84285714 -0.82857143 -0.81428571 -0.8 -0.78571429 -0.77142857 -0.75714286 -0.74285714 -0.72857143 -0.71428571 -0.7 -0.68571429 -0.67142857 -0.65714286 -0.64285714 -0.62857143 -0.61428571 -0.6 -0.58571429 -0.57142857 -0.55714286 -0.54285714 -0.52857143 -0.51428571 -0.5 -0.48571429 -0.47142857 -0.45714286 -0.44285714 -0.42857143 -0.41428571 -0.4 -0.38571429 -0.37142857 -0.35714286 -0.34285714 -0.32857143 -0.31428571 -0.3 -0.28571429 -0.27142857 -0.25714286 -0.24285714 -0.22857143 -0.21428571 -0.2 -0.18571429 -0.17142857 -0.15714286 -0.14285714 -0.12857143 -0.11428571 -0.1 -0.08571429 -0.07142857 -0.05714286 -0.04285714 -0.02857143 -0.01428571 0 0 0 0 0 0
  line L91 (2.7933, -13.3998) -> (2.7808, -13.4672)
  arc A175 (2.4999, -13.669) -> (2.7808, -13.4672) centre (2.535, -13.4215) ccw
  arc A176 (2.4999, -13.669) -> (2.3857, -13.6539) centre (1.6741, -19.5) ccw
  arc A177 (2.1666, -13.3863) -> (2.3857, -13.6539) centre (2.4159, -13.4058) ccw
  line L92 (2.1666, -13.3863) -> (2.172, -13.318)
  spline S84 degree 5 poles (2.172, -13.318) (2.1722, -13.3153) (2.1725, -13.3098) (2.1729, -13.3016) (2.173, -13.2906) (2.1725, -13.2768) (2.1717, -13.2631) (2.1707, -13.2493) (2.1695, -13.2355) (2.1682, -13.2217) (2.1668, -13.2079) (2.1653, -13.194) (2.1637, -13.1802) (2.1618, -13.1664) (2.1598, -13.1525) (2.1576, -13.1387) (2.1553, -13.1248) (2.1528, -13.111) (2.1502, -13.0971) (2.1475, -13.0832) (2.1447, -13.0694) (2.1418, -13.0555) (2.1388, -13.0417) (2.1356, -13.0278) (2.1324, -13.0139) (2.129, -13.0001) (2.1255, -12.9862) (2.1219, -12.9723) (2.1182, -12.9585) (2.1145, -12.9446) (2.1106, -12.9307) (2.1066, -12.9169) (2.1025, -12.903) (2.0984, -12.8891) (2.0941, -12.8753) (2.0898, -12.8614) (2.0853, -12.8476) (2.0808, -12.8337) (2.0762, -12.8199) (2.0715, -12.806) (2.0667, -12.7922) (2.0618, -12.7784) (2.0568, -12.7645) (2.0518, -12.7507) (2.0466, -12.7369) (2.0414, -12.7231) (2.0361, -12.7093) (2.0307, -12.6955) (2.0253, -12.6817) (2.0197, -12.6679) (2.0141, -12.6541) (2.0084, -12.6403) (2.0026, -12.6265) (1.9967, -12.6128) (1.9908, -12.599) (1.9847, -12.5853) (1.9786, -12.5715) (1.9725, -12.5578) (1.9662, -12.544) (1.9599, -12.5303) (1.9535, -12.5166) (1.947, -12.5029) (1.9404, -12.4892) (1.9338, -12.4755) (1.9271, -12.4618) (1.9203, -12.4481) (1.9135, -12.4345) (1.9066, -12.4208) (1.8996, -12.4072) (1.8925, -12.3936) (1.8854, -12.3799) (1.8796, -12.369) (1.8753, -12.3609) (1.8724, -12.3554) (1.8709, -12.3527) knots 0 0 0 0 0 0 0.01428571 0.02857143 0.04285714 0.05714286 0.07142857 0.08571429 0.1 0.11428571 0.12857143 0.14285714 0.15714286 0.17142857 0.18571429 0.2 0.21428571 0.22857143 0.24285714 0.25714286 0.27142857 0.28571429 0.3 0.31428571 0.32857143 0.34285714 0.35714286 0.37142857 0.38571429 0.4 0.41428571 0.42857143 0.44285714 0.45714286 0.47142857 0.48571429 0.5 0.51428571 0.52857143 0.54285714 0.55714286 0.57142857 0.58571429 0.6 0.61428571 0.62857143 0.64285714 0.65714286 0.67142857 0.68571429 0.7 0.71428571 0.72857143 0.74285714 0.75714286 0.77142857 0.78571429 0.8 0.81428571 0.82857143 0.84285714 0.85714286 0.87142857 0.88571429 0.9 0.91428571 0.92857143 0.94285714 0.95714286 0.97142857 0.98571429 1 1 1 1 1 1
  arc A178 (1.8709, -12.3527) -> (1.4774, -12.3527) centre (1.6741, -19.5) ccw
  spline S85 degree 5 poles (1.4774, -12.3527) (1.4759, -12.3554) (1.473, -12.3609) (1.4687, -12.369) (1.4629, -12.3799) (1.4558, -12.3936) (1.4487, -12.4072) (1.4417, -12.4208) (1.4348, -12.4345) (1.4279, -12.4481) (1.4212, -12.4618) (1.4145, -12.4755) (1.4078, -12.4892) (1.4013, -12.5029) (1.3948, -12.5166) (1.3884, -12.5303) (1.3821, -12.544) (1.3758, -12.5578) (1.3696, -12.5715) (1.3635, -12.5853) (1.3575, -12.599) (1.3516, -12.6128) (1.3457, -12.6265) (1.3399, -12.6403) (1.3342, -12.6541) (1.3286, -12.6679) (1.323, -12.6817) (1.3176, -12.6955) (1.3122, -12.7093) (1.3069, -12.7231) (1.3016, -12.7369) (1.2965, -12.7507) (1.2915, -12.7645) (1.2865, -12.7784) (1.2816, -12.7922) (1.2768, -12.806) (1.2721, -12.8199) (1.2675, -12.8337) (1.2629, -12.8476) (1.2585, -12.8614) (1.2541, -12.8753) (1.2499, -12.8891) (1.2457, -12.903) (1.2417, -12.9169) (1.2377, -12.9307) (1.2338, -12.9446) (1.23, -12.9585) (1.2264, -12.9723) (1.2228, -12.9862) (1.2193, -13.0001) (1.2159, -13.0139) (1.2127, -13.0278) (1.2095, -13.0417) (1.2065, -13.0555) (1.2036, -13.0694) (1.2008, -13.0832) (1.1981, -13.0971) (1.1955, -13.111) (1.193, -13.1248) (1.1907, -13.1387) (1.1885, -13.1525) (1.1864, -13.1664) (1.1846, -13.1802) (1.183, -13.194) (1.1815, -13.2079) (1.1801, -13.2217) (1.1788, -13.2355) (1.1776, -13.2493) (1.1765, -13.2631) (1.1757, -13.2768) (1.1753, -13.2906) (1.1754, -13.3016) (1.1757, -13.3098) (1.1761, -13.3153) (1.1763, -13.318) knots -1 -1 -1 -1 -1 -1 -0.98571429 -0.97142857 -0.95714286 -0.94285714 -0.92857143 -0.91428571 -0.9 -0.88571429 -0.87142857 -0.85714286 -0.84285714 -0.82857143 -0.81428571 -0.8 -0.78571429 -0.77142857 -0.75714286 -0.74285714 -0.72857143 -0.71428571 -0.7 -0.68571429 -0.67142857 -0.65714286 -0.64285714 -0.62857143 -0.61428571 -0.6 -0.58571429 -0.57142857 -0.55714286 -0.54285714 -0.52857143 -0.51428571 -0.5 -0.48571429 -0.47142857 -0.45714286 -0.44285714 -0.42857143 -0.41428571 -0.4 -0.38571429 -0.37142857 -0.35714286 -0.34285714 -0.32857143 -0.31428571 -0.3 -0.28571429 -0.27142857 -0.25714286 -0.24285714 -0.22857143 -0.21428571 -0.2 -0.18571429 -0.17142857 -0.15714286 -0.14285714 -0.12857143 -0.11428571 -0.1 -0.08571429 -0.07142857 -0.05714286 -0.04285714 -0.02857143 -0.01428571 0 0 0 0 0 0
  line L93 (1.1763, -13.318) -> (1.1816, -13.3863)
  arc A179 (0.9626, -13.6539) -> (1.1816, -13.3863) centre (0.9324, -13.4058) ccw
  arc A180 (0.9626, -13.6539) -> (0.8484, -13.669) centre (1.6741, -19.5) ccw
  arc A181 (0.5675, -13.4672) -> (0.8484, -13.669) centre (0.8133, -13.4215) ccw
  line L94 (0.5675, -13.4672) -> (0.555, -13.3998)
  spline S86 degree 5 poles (0.555, -13.3998) (0.5545, -13.3971) (0.5534, -13.3917) (0.5516, -13.3837) (0.5488, -13.3731) (0.5449, -13.3599) (0.5405, -13.3468) (0.536, -13.3338) (0.5312, -13.3207) (0.5264, -13.3077) (0.5215, -13.2947) (0.5165, -13.2818) (0.5113, -13.2688) (0.5059, -13.256) (0.5004, -13.2431) (0.4947, -13.2303) (0.4888, -13.2175) (0.4829, -13.2048) (0.4768, -13.1921) (0.4706, -13.1794) (0.4643, -13.1667) (0.4579, -13.1541) (0.4514, -13.1415) (0.4448, -13.1289) (0.438, -13.1163) (0.4312, -13.1038) (0.4242, -13.0913) (0.4172, -13.0789) (0.41, -13.0664) (0.4028, -13.054) (0.3955, -13.0416) (0.388, -13.0292) (0.3805, -13.0169) (0.3729, -13.0046) (0.3652, -12.9923) (0.3574, -12.9801) (0.3496, -12.9678) (0.3416, -12.9556) (0.3335, -12.9435) (0.3254, -12.9313) (0.3172, -12.9192) (0.3089, -12.9071) (0.3005, -12.895) (0.2921, -12.883) (0.2835, -12.8709) (0.2749, -12.8589) (0.2662, -12.847) (0.2574, -12.835) (0.2486, -12.8231) (0.2396, -12.8112) (0.2306, -12.7994) (0.2216, -12.7875) (0.2124, -12.7757) (0.2032, -12.764) (0.1939, -12.7522) (0.1845, -12.7405) (0.175, -12.7288) (0.1655, -12.7171) (0.1559, -12.7055) (0.1463, -12.6938) (0.1365, -12.6823) (0.1267, -12.6707) (0.1168, -12.6592) (0.1069, -12.6476) (0.0969, -12.6362) (0.0868, -12.6247) (0.0767, -12.6133) (0.0664, -12.6019) (0.0562, -12.5905) (0.0458, -12.5792) (0.0354, -12.5679) (0.027, -12.5588) (0.0207, -12.5521) (0.0164, -12.5476) (0.0143, -12.5453) knots 0 0 0 0 0 0 0.01428571 0.02857143 0.04285714 0.05714286 0.07142857 0.08571429 0.1 0.11428571 0.12857143 0.14285714 0.15714286 0.17142857 0.18571429 0.2 0.21428571 0.22857143 0.24285714 0.25714286 0.27142857 0.28571429 0.3 0.31428571 0.32857143 0.34285714 0.35714286 0.37142857 0.38571429 0.4 0.41428571 0.42857143 0.44285714 0.45714286 0.47142857 0.48571429 0.5 0.51428571 0.52857143 0.54285714 0.55714286 0.57142857 0.58571429 0.6 0.61428571 0.62857143 0.64285714 0.65714286 0.67142857 0.68571429 0.7 0.71428571 0.72857143 0.74285714 0.75714286 0.77142857 0.78571429 0.8 0.81428571 0.82857143 0.84285714 0.85714286 0.87142857 0.88571429 0.9 0.91428571 0.92857143 0.94285714 0.95714286 0.97142857 0.98571429 1 1 1 1 1 1
  arc A182 (0.0143, -12.5453) -> (-0.3658, -12.6472) centre (1.6741, -19.5) ccw
  spline S87 degree 5 poles (-0.3658, -12.6472) (-0.3665, -12.6502) (-0.3679, -12.6562) (-0.37, -12.6652) (-0.3727, -12.6772) (-0.3761, -12.6922) (-0.3794, -12.7072) (-0.3826, -12.7222) (-0.3858, -12.7372) (-0.3888, -12.7522) (-0.3918, -12.7671) (-0.3948, -12.7821) (-0.3976, -12.797) (-0.4004, -12.8119) (-0.4031, -12.8269) (-0.4058, -12.8418) (-0.4083, -12.8567) (-0.4108, -12.8715) (-0.4132, -12.8864) (-0.4155, -12.9013) (-0.4178, -12.9161) (-0.42, -12.9309) (-0.4221, -12.9458) (-0.4241, -12.9606) (-0.4261, -12.9753) (-0.4279, -12.9901) (-0.4297, -13.0049) (-0.4314, -13.0196) (-0.4331, -13.0344) (-0.4346, -13.0491) (-0.4361, -13.0638) (-0.4375, -13.0784) (-0.4388, -13.0931) (-0.44, -13.1077) (-0.4411, -13.1224) (-0.4422, -13.137) (-0.4431, -13.1516) (-0.444, -13.1661) (-0.4448, -13.1807) (-0.4455, -13.1952) (-0.4461, -13.2097) (-0.4467, -13.2242) (-0.4471, -13.2387) (-0.4474, -13.2531) (-0.4477, -13.2675) (-0.4478, -13.2819) (-0.4479, -13.2963) (-0.4479, -13.3106) (-0.4477, -13.325) (-0.4475, -13.3393) (-0.4472, -13.3535) (-0.4467, -13.3678) (-0.4462, -13.382) (-0.4455, -13.3961) (-0.4447, -13.4103) (-0.4439, -13.4244) (-0.4429, -13.4385) (-0.4418, -13.4525) (-0.4406, -13.4666) (-0.4393, -13.4806) (-0.4378, -13.4945) (-0.4362, -13.5084) (-0.4344, -13.5222) (-0.4324, -13.536) (-0.4303, -13.5498) (-0.428, -13.5635) (-0.4257, -13.5771) (-0.4233, -13.5908) (-0.4207, -13.6044) (-0.4179, -13.6179) (-0.4148, -13.6313) (-0.4119, -13.6419) (-0.4094, -13.6497) (-0.4076, -13.6549) (-0.4067, -13.6575) knots -1 -1 -1 -1 -1 -1 -0.98571429 -0.97142857 -0.95714286 -0.94285714 -0.92857143 -0.91428571 -0.9 -0.88571429 -0.87142857 -0.85714286 -0.84285714 -0.82857143 -0.81428571 -0.8 -0.78571429 -0.77142857 -0.75714286 -0.74285714 -0.72857143 -0.71428571 -0.7 -0.68571429 -0.67142857 -0.65714286 -0.64285714 -0.62857143 -0.61428571 -0.6 -0.58571429 -0.57142857 -0.55714286 -0.54285714 -0.52857143 -0.51428571 -0.5 -0.48571429 -0.47142857 -0.45714286 -0.44285714 -0.42857143 -0.41428571 -0.4 -0.38571429 -0.37142857 -0.35714286 -0.34285714 -0.32857143 -0.31428571 -0.3 -0.28571429 -0.27142857 -0.25714286 -0.24285714 -0.22857143 -0.21428571 -0.2 -0.18571429 -0.17142857 -0.15714286 -0.14285714 -0.12857143 -0.11428571 -0.1 -0.08571429 -0.07142857 -0.05714286 -0.04285714 -0.02857143 -0.01428571 0 0 0 0 0 0
  line L95 (-0.4067, -13.6575) -> (-0.3839, -13.7221)
  arc A183 (-0.5262, -14.0373) -> (-0.3839, -13.7221) centre (-0.6196, -13.8054) ccw
  arc A184 (-0.5262, -14.0373) -> (-0.6327, -14.0814) centre (1.6741, -19.5) ccw
  arc A185 (-0.9562, -13.9592) -> (-0.6327, -14.0814) centre (-0.7306, -13.8514) ccw
  line L96 (-0.9562, -13.9592) -> (-0.9857, -13.8974)
  spline S88 degree 5 poles (-0.9857, -13.8974) (-0.9869, -13.8949) (-0.9893, -13.8899) (-0.9931, -13.8826) (-0.9986, -13.8731) (-1.0058, -13.8614) (-1.0134, -13.8499) (-1.0212, -13.8384) (-1.0291, -13.8271) (-1.0372, -13.8158) (-1.0453, -13.8045) (-1.0535, -13.7933) (-1.0618, -13.7821) (-1.0703, -13.7711) (-1.079, -13.7601) (-1.0878, -13.7492) (-1.0968, -13.7384) (-1.1059, -13.7276) (-1.115, -13.7169) (-1.1243, -13.7063) (-1.1337, -13.6957) (-1.1431, -13.6851) (-1.1527, -13.6746) (-1.1623, -13.6642) (-1.1721, -13.6538) (-1.1819, -13.6435) (-1.1919, -13.6332) (-1.2019, -13.623) (-1.212, -13.6128) (-1.2222, -13.6027) (-1.2325, -13.5926) (-1.2429, -13.5826) (-1.2533, -13.5726) (-1.2639, -13.5627) (-1.2745, -13.5528) (-1.2852, -13.543) (-1.296, -13.5332) (-1.3068, -13.5235) (-1.3177, -13.5138) (-1.3287, -13.5042) (-1.3398, -13.4946) (-1.351, -13.4851) (-1.3622, -13.4756) (-1.3735, -13.4661) (-1.3848, -13.4567) (-1.3962, -13.4474) (-1.4077, -13.4381) (-1.4193, -13.4288) (-1.431, -13.4196) (-1.4427, -13.4104) (-1.4544, -13.4013) (-1.4663, -13.3922) (-1.4782, -13.3832) (-1.4901, -13.3742) (-1.5022, -13.3653) (-1.5142, -13.3564) (-1.5264, -13.3475) (-1.5386, -13.3387) (-1.5509, -13.3299) (-1.5632, -13.3212) (-1.5756, -13.3125) (-1.5881, -13.3039) (-1.6006, -13.2953) (-1.6132, -13.2868) (-1.6259, -13.2783) (-1.6386, -13.2698) (-1.6513, -13.2614) (-1.6641, -13.253) (-1.677, -13.2447) (-1.69, -13.2364) (-1.7029, -13.2282) (-1.7134, -13.2217) (-1.7212, -13.2168) (-1.7265, -13.2135) (-1.7291, -13.2119) knots 0 0 0 0 0 0 0.01428571 0.02857143 0.04285714 0.05714286 0.07142857 0.08571429 0.1 0.11428571 0.12857143 0.14285714 0.15714286 0.17142857 0.18571429 0.2 0.21428571 0.22857143 0.24285714 0.25714286 0.27142857 0.28571429 0.3 0.31428571 0.32857143 0.34285714 0.35714286 0.37142857 0.38571429 0.4 0.41428571 0.42857143 0.44285714 0.45714286 0.47142857 0.48571429 0.5 0.51428571 0.52857143 0.54285714 0.55714286 0.57142857 0.58571429 0.6 0.61428571 0.62857143 0.64285714 0.65714286 0.67142857 0.68571429 0.7 0.71428571 0.72857143 0.74285714 0.75714286 0.77142857 0.78571429 0.8 0.81428571 0.82857143 0.84285714 0.85714286 0.87142857 0.88571429 0.9 0.91428571 0.92857143 0.94285714 0.95714286 0.97142857 0.98571429 1 1 1 1 1 1
  arc A186 (-1.7291, -13.2119) -> (-2.0699, -13.4086) centre (1.6741, -19.5) ccw